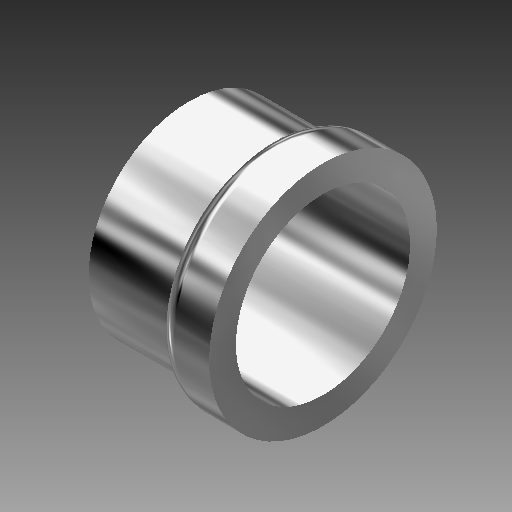
# Autodesk Inventor part: 405-03
Saved by Autodesk Inventor 2019 (Build 230136000, 136)
## iProperties
Company: Autodesk Inc.
Created: 2017-06-27
Part Number: 405-03
Material: Steel, Mild
Document SubType Name: Modeling
Designer: Autodesk Inc.
Mass: 4.87548 g
Surface Area: 10.6202 cm^2
Volume: 0.621081 cm^3
Density: 7.85 g/cm^3
Appearance: Chrome - Polished
Author: Inventor
Autodesk Inventor part; units mm, degrees
ref_plane "YZ Plane" through (0, 0, 0) normal (1, 0, 0) x (0, 1, 0)
ref_plane "XZ Plane" through (0, 0, 0) normal (0, 1, 0) x (-1, 0, 0)
ref_plane "XY Plane" through (0, 0, 0) normal (0, 0, 1) x (1, 0, 0)
sketch "Sketch1" plane through (0, 0, 0) normal (0, 0, 1) x (1, 0, 0)
  line L0 (0, 0) -> (6, 0)
  line L1 (6, 0) -> (6, 7.5)
  line L2 (6, 7.5) -> (0, 7.5)
  line L3 (0, 7.5) -> (0, 0)
  line L4 (6, 0) -> (10, 0)
  line L5 (10, 0) -> (10, 8.5)
  line L6 (10, 8.5) -> (6, 8.5)
  line L7 (6, 8.5) -> (6, 0)
  dimension "d0" = 15
  dimension "d1" = 17
  dimension "d2" = 6
  dimension "d3" = 10
  constraints: 16 end point, 4 parallel, 2 horizontal, 2 perpendicular
  measures "d0" diameter of L2 L0
  measures "d1" diameter of L6 L4
  measures "d2" distance of L1.end L2.end
  measures "d3" distance between parallel lines of L5 L3
revolve "Revolution1" add sketch "Sketch1" angle 360 about axis through (0, 0, 0) along (1, 0, 0)
fillet "Fillet1" radius 1.5 1 edges at (6, -8.5, 0)
hole "Hole1" at (10, 0, 0) direction (-1, 0, 0) diameter 13 end through all
body "Solid1"
